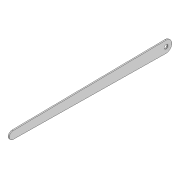
# Autodesk Inventor part: BrazoPalanca
Saved by Autodesk Inventor 2021 (Build 250183000, 183)
## iProperties
Created: 2021-05-09
Part Number: BrazoPalanca
Material: Genérico
Document SubType Name: Modeling
Designer: carlo
Density: 1 g/cm^3
Appearance: Valor por defecto
Author: carlo
Autodesk Inventor part; units mm, degrees
ref_plane "YZ Plane" through (0, 0, 0) normal (1, 0, 0) x (0, 1, 0)
ref_plane "XZ Plane" through (0, 0, 0) normal (0, 1, 0) x (-1, 0, 0)
ref_plane "XY Plane" through (0, 0, 0) normal (0, 0, 1) x (1, 0, 0)
sketch "Boceto1" plane through (0, 0, -197.5) normal (1, 0, 0) x (0, 1, 0)
  arc A0 (10, 400) -> (-10, 400) centre (0, 400) ccw
  line L0 (-10, 400) -> (-15, 0)
  line L1 (10, 400) -> (15, 0)
  arc A1 (-14.9953, 0.3749) -> (14.9953, 0.3749) centre (0, 0) ccw
  circle A2 centre (0, 0) radius 5
  dimension "d1" = 20
  dimension "d0" = 10
  constraints: 5 point on circle, 4 end point, 3 centre point, 2 point on line, 1 coincident
  measures "d1" diameter of A0
  measures "d0" diameter of A2
extrude "Extrusión1" add sketch "Boceto1" along normal blind 3
